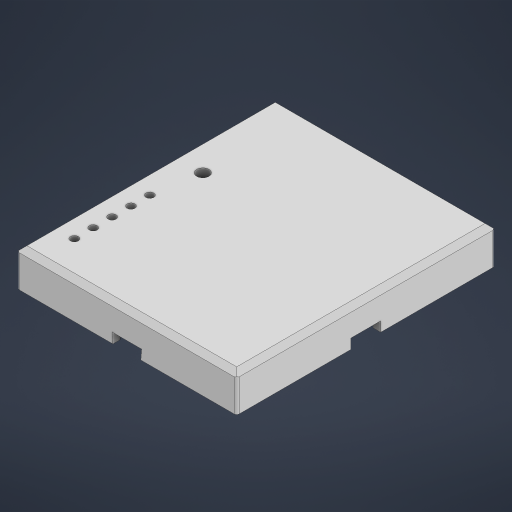
# Autodesk Inventor part: enclosure3_top
Saved by Autodesk Inventor 2023 (Build 270158000, 158)
## iProperties
Created: 2022-05-05
Part Number: enclosure3_top
Material: Generic
Document SubType Name: Modeling
Designer: Haroon Nawaz
Density: 1 g/cm^3
Appearance: Default
Author: Haroon Nawaz
Autodesk Inventor part; units mm, degrees
note: some values were not read from the file. Chosen so that the rebuilt part matches the saved one: direction of "Emboss2".
ref_plane "YZ Plane" through (0, 0, 0) normal (1, 0, 0) x (0, 1, 0)
ref_plane "XZ Plane" through (0, 0, 0) normal (0, 1, 0) x (-1, 0, 0)
ref_plane "XY Plane" through (0, 0, 0) normal (0, 0, 1) x (1, 0, 0)
sketch "Sketch1" plane through (0, 0, 0) normal (0, 1, 0) x (-1, 0, 0)
  line L0 (0, 0) -> (44.4, 0)
  line L1 (44.4, 0) -> (44.4, -52.2)
  line L2 (44.4, -52.2) -> (0, -52.2)
  line L3 (0, -52.2) -> (0, 0)
  dimension "d2" = 44.4
  dimension "d3" = 52.2
  constraints: 8 end point, 2 parallel, 1 horizontal, 1 perpendicular
  measures "d2" distance of L1.end L2.end
  measures "d3" distance of L0.end L1.end
extrude "Extrusion1" add sketch "Sketch1" along normal blind 7.5
shell "Shell1" thickness 1.5 removed faces 1 at (-14.8, 0, -17.4)
chamfer "Chamfer1" distance 1 angle 45 5 edges at (0, 7.5, -26.1) (-22.2, 7.5, 0) (-22.2, 7.5, -52.2) (-44.4, 7.5, -26.1) (-42.9, 3, -50.7)
sketch "Sketch3" plane through (0, 7.5, 0) normal (0, 1, 0) x (1, 0, 0)
  line L0 (-44.4, 52.2) -> (-44.4, 31.531)
  line L1 (-44.4, 52.2) -> (-44.4, 0) projected
  line L2 (-44.4, 31.531) -> (-38.38, 31.531)
  point P0 (0, 0)
  point P1 (-44.4, 51.45)
  point P2 (-44.4, 0.75)
  dimension "d26" = 20.669
  dimension "d27" = 6.02
  constraints: 4 end point, 1 coincident, 1 horizontal, 1 point on line
  measures "d26" distance of L0.start L0.end
  measures "d27" distance of L0.end L2.end
hole "Hole1" at (-38.38, 7.5, -31.531) direction (0, -1, 0) diameter 2.5 depth 3 tip angle 118
fillet "Fillet1" radius 0.5 4 edges at (0, 3.25, -52.2) (0, 3.25, 0) (-44.4, 3.25, -52.2) (-44.4, 3.25, 0)
sketch "Sketch4" plane through (-1.5, 6, -50.7) normal (0, -1, 0) x (1, 0, 0)
  circle A0 centre (-36.88, 19.169) radius 1.25 projected
  circle A1 centre (-36.88, 19.169) radius 1.5
  circle A2 centre (-36.88, 19.169) radius 1.125
  point P0 (1.5, 50.7)
  dimension "d36" = 3
  dimension "d40" = 2.25
  constraints: 2 centre point, 2 coincident
  measures "d36" diameter of A1
  measures "d40" diameter of A2
extrude "Extrusion3" add sketch "Sketch4" along normal blind 2.4 contours A1
fillet "Fillet2" radius 0.5 1 edges at (-39.88, 6, -31.531)
sketch "Sketch5" plane through (0, 7.5, 0) normal (0, 1, 0) x (1, 0, 0)
  line L0 (-44.3114, 52.075) -> (-44.3114, 22.635)
  line L1 (-44.4, 51.7) -> (-44.4, 0.5) projected
  line L2 (-44.3114, 52.075) -> (-14.8714, 52.075) construction
  line L3 (0, 0.5) -> (0, 51.7) projected
  point P0 (0, 0)
  point P1 (-44.4, 0)
  point P2 (-39.8266, 22.26)
  point P3 (-39.8266, 18.45)
  point P4 (-39.8266, 14.64)
  point P5 (-39.8266, 10.83)
  point P6 (-39.8266, 7.02)
  dimension "d41" = 29.44
  dimension "d42" = 90
  dimension "d46" = 3.81
  dimension "d58" = 4.5734
  dimension "d81" = 39.8266
  constraints: 4 end point, 1 horizontal, 1 parallel, 1 perpendicular, 1 vertical, 4 other
  measures "d41" distance of L0.start L0.end
  measures "d42" angle of L0 L2
  measures "d46" distance of point (-39.827, 22.26) point (-39.827, 18.45)
  measures "d58" distance from line of L1 point (-39.827, 22.26)
  measures "d81" distance from line of point (-39.827, 22.26) L3
hole "Hole2" at (-39.8266, 7.5, -22.26) at (-39.8266, 7.5, -18.45) at (-39.8266, 7.5, -14.64) at (-39.8266, 7.5, -10.83) at (-39.8266, 7.5, -7.02) direction (0, -1, 0) diameter 1.6 depth 3 tip angle 118
sketch "Sketch6" plane through (-0.5, 0, -52.2) normal (0, 0, -1) x (-1, 0, 0)
  line L0 (-0.5, 0) -> (1.82, 0)
  line L1 (-0.5, 0) -> (33.3, 0)
  line L2 (42.4, 0) -> (1, 0) projected
  line L3 (1.82, 0) -> (33.3, 0)
  line L4 (33.3, 0) -> (33.3, 3.175)
  line L5 (33.3, 3.175) -> (1.82, 3.175)
  line L6 (1.82, 3.175) -> (1.82, 0)
  point P0 (41.9, 0)
  dimension "d59" = 2.32
  dimension "d60" = 33.8
  dimension "d61" = 3.175
  constraints: 12 end point, 2 horizontal, 2 parallel, 1 perpendicular, 1 point on line
  measures "d59" distance of L0.start L0.end
  measures "d60" distance of L0.start L1.end
  measures "d61" distance of L3.end L4.end
extrude "Extrusion4" cut sketch "Sketch6" against normal blind 1.5
sketch "Sketch8" plane through (-1.5, 6, -50.7) normal (0, -1, 0) x (1, 0, 0)
  line L0 (-18.1366, 47.9399) -> (24.8957, 47.9399) construction
  line L1 (24.8957, 47.9399) -> (24.8957, 43.6819) construction
  line L2 (24.8957, 43.6819) -> (-18.1366, 43.6819) construction
  line L3 (-18.1366, 43.6819) -> (-18.1366, 47.9399) construction
  line L4 (-16.6442, 44.4831) -> (-18.0503, 44.4831)
  line L5 (-18.0503, 44.4831) -> (-18.0503, 44.6455)
  spline S0 degree 2 poles (-18.0503, 44.6455) (-17.9919, 44.6506) (-17.8828, 44.6633) (-17.8396, 44.6785) knots 0 0 0 1 2 2 2
  spline S1 degree 2 poles (-17.8396, 44.6785) (-17.766, 44.7064) (-17.7152, 44.8054) (-17.7152, 44.8891) knots 0 0 0 1 2 2 2
  line L6 (-17.7152, 44.8891) -> (-17.7152, 47.3637)
  spline S2 degree 2 poles (-17.7152, 47.3637) (-17.7152, 47.45) (-17.7838, 47.5947) (-17.8421, 47.6328) knots 0 0 0 1 2 2 2
  spline S3 degree 2 poles (-17.8421, 47.6328) (-17.8878, 47.6607) (-18.068, 47.714) (-18.1366, 47.7191) knots 0 0 0 1 2 2 2
  line L7 (-18.1366, 47.7191) -> (-18.1366, 47.8815)
  line L8 (-18.1366, 47.8815) -> (-17.0122, 47.9399)
  line L9 (-17.0122, 47.9399) -> (-16.9792, 47.9043)
  line L10 (-16.9792, 47.9043) -> (-16.9792, 44.9171)
  spline S4 degree 2 poles (-16.9792, 44.9171) (-16.9792, 44.8358) (-16.9208, 44.7318) (-16.8549, 44.7039) knots 0 0 0 1 2 2 2
  spline S5 degree 2 poles (-16.8549, 44.7039) (-16.8117, 44.6836) (-16.7127, 44.6531) (-16.6442, 44.6455) knots 0 0 0 1 2 2 2
  line L11 (-16.6442, 44.6455) -> (-16.6442, 44.4831)
  spline S6 degree 2 poles (-14.0326, 45.0186) (-14.1112, 44.8891) (-14.332, 44.6633) (-14.4716, 44.5846) knots 0 0 0 1 2 2 2
  spline S7 degree 2 poles (-14.4716, 44.5846) (-14.6214, 44.4983) (-14.9285, 44.412) (-15.1265, 44.412) knots 0 0 0 1 2 2 2
  spline S8 degree 2 poles (-15.1265, 44.412) (-15.4589, 44.412) (-15.9386, 44.5998) (-16.096, 44.7572) knots 0 0 0 1 2 2 2
  spline S9 degree 2 poles (-16.096, 44.7572) (-16.2508, 44.9171) (-16.4056, 45.3485) (-16.4056, 45.5998) knots 0 0 0 1 2 2 2
  spline S10 degree 2 poles (-16.4056, 45.5998) (-16.4056, 45.8282) (-16.2381, 46.247) (-16.0833, 46.4094) knots 0 0 0 1 2 2 2
  spline S11 degree 2 poles (-16.0833, 46.4094) (-15.931, 46.5693) (-15.4691, 46.7648) (-15.1848, 46.7648) knots 0 0 0 1 2 2 2
  spline S12 degree 2 poles (-15.1848, 46.7648) (-14.8701, 46.7648) (-14.4691, 46.6125) (-14.3371, 46.478) knots 0 0 0 1 2 2 2
  spline S13 degree 2 poles (-14.3371, 46.478) (-14.2102, 46.3511) (-14.0935, 46.0059) (-14.0935, 45.8155) knots 0 0 0 1 2 2 2
  line L12 (-14.0935, 45.8155) -> (-14.0935, 45.6709)
  line L13 (-14.0935, 45.6709) -> (-15.6036, 45.6709)
  spline S14 degree 2 poles (-15.6036, 45.6709) (-15.6036, 45.2115) (-15.2508, 44.7343) (-14.865, 44.7343) knots 0 0 0 1 2 2 2
  spline S15 degree 2 poles (-14.865, 44.7343) (-14.6569, 44.7343) (-14.3219, 44.9653) (-14.2026, 45.1404) knots 0 0 0 1 2 2 2
  line L14 (-14.2026, 45.1404) -> (-14.0326, 45.0186)
  spline S16 degree 2 poles (-14.8853, 45.8688) (-14.8853, 46.0008) (-14.9133, 46.2825) (-14.9463, 46.3714) knots 0 0 0 1 2 2 2
  spline S17 degree 2 poles (-14.9463, 46.3714) (-14.9843, 46.478) (-15.1163, 46.5846) (-15.2153, 46.5846) knots 0 0 0 1 2 2 2
  spline S18 degree 2 poles (-15.2153, 46.5846) (-15.3879, 46.5846) (-15.5934, 46.2368) (-15.6036, 45.8587) knots 0 0 0 1 2 2 2
  line L15 (-15.6036, 45.8587) -> (-14.8853, 45.8688)
  line L16 (-10.157, 46.445) -> (-10.6494, 46.445)
  spline S19 degree 2 poles (-10.6494, 46.445) (-10.5605, 46.3485) (-10.4742, 46.1302) (-10.4742, 46.011) knots 0 0 0 1 2 2 2
  spline S20 degree 2 poles (-10.4742, 46.011) (-10.4742, 45.8587) (-10.6392, 45.5871) (-10.7737, 45.5033) knots 0 0 0 1 2 2 2
  spline S21 degree 2 poles (-10.7737, 45.5033) (-10.9082, 45.4171) (-11.2763, 45.3181) (-11.4895, 45.3181) knots 0 0 0 1 2 2 2
  line L17 (-11.4895, 45.3181) -> (-11.8549, 45.3181)
  spline S22 degree 2 poles (-11.8549, 45.3181) (-11.8803, 45.2978) (-11.9463, 45.2115) (-11.9463, 45.1709) knots 0 0 0 1 2 2 2
  spline S23 degree 2 poles (-11.9463, 45.1709) (-11.9463, 45.0719) (-11.7889, 44.9957) (-11.5834, 44.9907) knots 0 0 0 1 2 2 2
  spline S24 degree 2 poles (-11.5834, 44.9907) (-11.3803, 44.9856) (-10.9666, 44.9627) (-10.8778, 44.9602) knots 0 0 0 1 2 2 2
  spline S25 degree 2 poles (-10.8778, 44.9602) (-10.7483, 44.9526) (-10.492, 44.8612) (-10.3981, 44.7876) knots 0 0 0 1 2 2 2
  spline S26 degree 2 poles (-10.3981, 44.7876) (-10.2966, 44.7089) (-10.1621, 44.4653) (-10.1621, 44.3079) knots 0 0 0 1 2 2 2
  spline S27 degree 2 poles (-10.1621, 44.3079) (-10.1621, 44.1379) (-10.3245, 43.8384) (-10.492, 43.7293) knots 0 0 0 1 2 2 2
  spline S28 degree 2 poles (-10.492, 43.7293) (-10.6697, 43.6151) (-11.162, 43.4907) (-11.525, 43.4907) knots 0 0 0 1 2 2 2
  spline S29 degree 2 poles (-11.525, 43.4907) (-12.1113, 43.4907) (-12.7229, 43.7775) (-12.7229, 44.0617) knots 0 0 0 1 2 2 2
  spline S30 degree 2 poles (-12.7229, 44.0617) (-12.7229, 44.2394) (-12.393, 44.4678) (-12.0478, 44.478) knots 0 0 0 1 2 2 2
  line L18 (-12.0478, 44.478) -> (-12.0478, 44.5059)
  spline S31 degree 2 poles (-12.0478, 44.5059) (-12.2534, 44.5744) (-12.4818, 44.8029) (-12.4818, 44.9551) knots 0 0 0 1 2 2 2
  spline S32 degree 2 poles (-12.4818, 44.9551) (-12.4818, 45.049) (-12.3905, 45.1785) (-12.3194, 45.2292) knots 0 0 0 1 2 2 2
  spline S33 degree 2 poles (-12.3194, 45.2292) (-12.2559, 45.2699) (-12.0757, 45.3308) (-12.0174, 45.3485) knots 0 0 0 1 2 2 2
  line L19 (-12.0174, 45.3485) -> (-12.0174, 45.3739)
  spline S34 degree 2 poles (-12.0174, 45.3739) (-12.3169, 45.4856) (-12.6011, 45.8079) (-12.6011, 46.0389) knots 0 0 0 1 2 2 2
  spline S35 degree 2 poles (-12.6011, 46.0389) (-12.6011, 46.3663) (-11.9971, 46.7597) (-11.5326, 46.7597) knots 0 0 0 1 2 2 2
  spline S36 degree 2 poles (-11.5326, 46.7597) (-11.3803, 46.7597) (-11.0961, 46.7089) (-11.0225, 46.6886) knots 0 0 0 1 2 2 2
  line L20 (-11.0225, 46.6886) -> (-10.157, 46.6886)
  line L21 (-10.157, 46.6886) -> (-10.157, 46.445)
  spline S37 degree 2 poles (-10.8321, 44.1455) (-10.8321, 44.2216) (-10.9159, 44.3714) (-11.0631, 44.4171) knots 0 0 0 1 2 2 2
  spline S38 degree 2 poles (-11.0631, 44.4171) (-11.1443, 44.4298) (-11.5098, 44.4399) (-11.8296, 44.4399) knots 0 0 0 1 2 2 2
  spline S39 degree 2 poles (-11.8296, 44.4399) (-11.9082, 44.3739) (-12.0123, 44.1886) (-12.0123, 44.0592) knots 0 0 0 1 2 2 2
  spline S40 degree 2 poles (-12.0123, 44.0592) (-12.0123, 44.0034) (-11.9488, 43.8689) (-11.8828, 43.813) knots 0 0 0 1 2 2 2
  spline S41 degree 2 poles (-11.8828, 43.813) (-11.8067, 43.747) (-11.6138, 43.6734) (-11.4209, 43.6734) knots 0 0 0 1 2 2 2
  spline S42 degree 2 poles (-11.4209, 43.6734) (-11.1341, 43.6734) (-10.8321, 43.8968) (-10.8321, 44.1455) knots 0 0 0 1 2 2 2
  spline S43 degree 2 poles (-11.2052, 46.0211) (-11.2052, 46.2825) (-11.3702, 46.5846) (-11.5428, 46.5846) knots 0 0 0 1 2 2 2
  spline S44 degree 2 poles (-11.5428, 46.5846) (-11.629, 46.5846) (-11.761, 46.5033) (-11.7991, 46.4247) knots 0 0 0 1 2 2 2
  spline S45 degree 2 poles (-11.7991, 46.4247) (-11.8372, 46.3485) (-11.8651, 46.1455) (-11.8651, 46.0389) knots 0 0 0 1 2 2 2
  spline S46 degree 2 poles (-11.8651, 46.0389) (-11.8651, 45.7952) (-11.695, 45.483) (-11.5377, 45.483) knots 0 0 0 1 2 2 2
  spline S47 degree 2 poles (-11.5377, 45.483) (-11.3778, 45.483) (-11.2052, 45.7648) (-11.2052, 46.0211) knots 0 0 0 1 2 2 2
  spline S48 degree 2 poles (-7.619, 45.0186) (-7.6976, 44.8891) (-7.9184, 44.6633) (-8.058, 44.5846) knots 0 0 0 1 2 2 2
  spline S49 degree 2 poles (-8.058, 44.5846) (-8.2078, 44.4983) (-8.5149, 44.412) (-8.7128, 44.412) knots 0 0 0 1 2 2 2
  spline S50 degree 2 poles (-8.7128, 44.412) (-9.0453, 44.412) (-9.525, 44.5998) (-9.6824, 44.7572) knots 0 0 0 1 2 2 2
  spline S51 degree 2 poles (-9.6824, 44.7572) (-9.8372, 44.9171) (-9.992, 45.3485) (-9.992, 45.5998) knots 0 0 0 1 2 2 2
  spline S52 degree 2 poles (-9.992, 45.5998) (-9.992, 45.8282) (-9.8245, 46.247) (-9.6697, 46.4094) knots 0 0 0 1 2 2 2
  spline S53 degree 2 poles (-9.6697, 46.4094) (-9.5174, 46.5693) (-9.0555, 46.7648) (-8.7712, 46.7648) knots 0 0 0 1 2 2 2
  spline S54 degree 2 poles (-8.7712, 46.7648) (-8.4565, 46.7648) (-8.0555, 46.6125) (-7.9235, 46.478) knots 0 0 0 1 2 2 2
  spline S55 degree 2 poles (-7.9235, 46.478) (-7.7966, 46.3511) (-7.6799, 46.0059) (-7.6799, 45.8155) knots 0 0 0 1 2 2 2
  line L22 (-7.6799, 45.8155) -> (-7.6799, 45.6709)
  line L23 (-7.6799, 45.6709) -> (-9.19, 45.6709)
  spline S56 degree 2 poles (-9.19, 45.6709) (-9.19, 45.2115) (-8.8372, 44.7343) (-8.4514, 44.7343) knots 0 0 0 1 2 2 2
  spline S57 degree 2 poles (-8.4514, 44.7343) (-8.2433, 44.7343) (-7.9083, 44.9653) (-7.789, 45.1404) knots 0 0 0 1 2 2 2
  line L24 (-7.789, 45.1404) -> (-7.619, 45.0186)
  spline S58 degree 2 poles (-8.4717, 45.8688) (-8.4717, 46.0008) (-8.4997, 46.2825) (-8.5326, 46.3714) knots 0 0 0 1 2 2 2
  spline S59 degree 2 poles (-8.5326, 46.3714) (-8.5707, 46.478) (-8.7027, 46.5846) (-8.8017, 46.5846) knots 0 0 0 1 2 2 2
  spline S60 degree 2 poles (-8.8017, 46.5846) (-8.9743, 46.5846) (-9.1798, 46.2368) (-9.19, 45.8587) knots 0 0 0 1 2 2 2
  line L25 (-9.19, 45.8587) -> (-8.4717, 45.8688)
  spline S61 degree 2 poles (-6.3702, 44.4069) (-6.5885, 44.4069) (-7.0022, 44.5364) (-7.1164, 44.6074) knots 0 0 0 1 2 2 2
  line L26 (-7.1164, 44.6074) -> (-7.1824, 44.4551)
  line L27 (-7.1824, 44.4551) -> (-7.3575, 44.4551)
  line L28 (-7.3575, 44.4551) -> (-7.3855, 45.2876)
  line L29 (-7.3855, 45.2876) -> (-7.223, 45.2876)
  spline S62 degree 2 poles (-7.223, 45.2876) (-7.19, 45.1861) (-7.0327, 44.9348) (-6.9312, 44.8333) knots 0 0 0 1 2 2 2
  spline S63 degree 2 poles (-6.9312, 44.8333) (-6.8271, 44.7343) (-6.5555, 44.5947) (-6.4032, 44.5947) knots 0 0 0 1 2 2 2
  spline S64 degree 2 poles (-6.4032, 44.5947) (-6.1977, 44.5947) (-5.9997, 44.7521) (-5.9997, 44.9196) knots 0 0 0 1 2 2 2
  spline S65 degree 2 poles (-5.9997, 44.9196) (-5.9997, 45.0084) (-6.0885, 45.1252) (-6.1672, 45.1658) knots 0 0 0 1 2 2 2
  spline S66 degree 2 poles (-6.1672, 45.1658) (-6.2535, 45.2115) (-6.4616, 45.2749) (-6.6139, 45.3181) knots 0 0 0 1 2 2 2
  spline S67 degree 2 poles (-6.6139, 45.3181) (-6.7662, 45.3638) (-6.9819, 45.4551) (-7.0987, 45.5541) knots 0 0 0 1 2 2 2
  spline S68 degree 2 poles (-7.0987, 45.5541) (-7.1976, 45.6404) (-7.3195, 45.8866) (-7.3195, 46.0566) knots 0 0 0 1 2 2 2
  spline S69 degree 2 poles (-7.3195, 46.0566) (-7.3195, 46.3714) (-6.7916, 46.7597) (-6.3626, 46.7597) knots 0 0 0 1 2 2 2
  spline S70 degree 2 poles (-6.3626, 46.7597) (-6.1596, 46.7597) (-5.817, 46.6759) (-5.7002, 46.6277) knots 0 0 0 1 2 2 2
  line L30 (-5.7002, 46.6277) -> (-5.6545, 46.7597)
  line L31 (-5.6545, 46.7597) -> (-5.4845, 46.7597)
  line L32 (-5.4845, 46.7597) -> (-5.4489, 45.9983)
  line L33 (-5.4489, 45.9983) -> (-5.6063, 45.9983)
  spline S71 degree 2 poles (-5.6063, 45.9983) (-5.685, 46.2292) (-6.0631, 46.5668) (-6.2814, 46.5668) knots 0 0 0 1 2 2 2
  spline S72 degree 2 poles (-6.2814, 46.5668) (-6.454, 46.5668) (-6.6494, 46.4247) (-6.6494, 46.2978) knots 0 0 0 1 2 2 2
  spline S73 degree 2 poles (-6.6494, 46.2978) (-6.6494, 46.1277) (-6.3626, 45.9754) (-6.1038, 45.9094) knots 0 0 0 1 2 2 2
  spline S74 degree 2 poles (-6.1038, 45.9094) (-5.7053, 45.8054) (-5.3347, 45.4501) (-5.3347, 45.1759) knots 0 0 0 1 2 2 2
  spline S75 degree 2 poles (-5.3347, 45.1759) (-5.3347, 44.8079) (-5.9083, 44.4069) (-6.3702, 44.4069) knots 0 0 0 1 2 2 2
  spline S76 degree 2 poles (-3.4008, 44.5846) (-3.5429, 44.5237) (-3.8703, 44.4221) (-4.1038, 44.4221) knots 0 0 0 1 2 2 2
  spline S77 degree 2 poles (-4.1038, 44.4221) (-4.4515, 44.4221) (-4.7891, 44.7622) (-4.7891, 45.0744) knots 0 0 0 1 2 2 2
  line L34 (-4.7891, 45.0744) -> (-4.7891, 46.445)
  line L35 (-4.7891, 46.445) -> (-5.1901, 46.445)
  line L36 (-5.1901, 46.445) -> (-5.1901, 46.6886)
  line L37 (-5.1901, 46.6886) -> (-4.7789, 46.6886)
  line L38 (-4.7789, 46.6886) -> (-4.7789, 47.3663)
  line L39 (-4.7789, 47.3663) -> (-4.0581, 47.3663)
  line L40 (-4.0581, 47.3663) -> (-4.0581, 46.6886)
  line L41 (-4.0581, 46.6886) -> (-3.4287, 46.6886)
  line L42 (-3.4287, 46.6886) -> (-3.4287, 46.445)
  line L43 (-3.4287, 46.445) -> (-4.053, 46.445)
  line L44 (-4.053, 46.445) -> (-4.053, 45.2242)
  spline S78 degree 2 poles (-4.053, 45.2242) (-4.053, 44.9627) (-3.9084, 44.7445) (-3.718, 44.7445) knots 0 0 0 1 2 2 2
  spline S79 degree 2 poles (-3.718, 44.7445) (-3.6596, 44.7445) (-3.4439, 44.7622) (-3.4008, 44.7724) knots 0 0 0 1 2 2 2
  line L45 (-3.4008, 44.7724) -> (-3.4008, 44.5846)
  spline S80 degree 2 poles (-0.8424, 45.0186) (-0.9211, 44.8891) (-1.1419, 44.6633) (-1.2815, 44.5846) knots 0 0 0 1 2 2 2
  spline S81 degree 2 poles (-1.2815, 44.5846) (-1.4312, 44.4983) (-1.7383, 44.412) (-1.9363, 44.412) knots 0 0 0 1 2 2 2
  spline S82 degree 2 poles (-1.9363, 44.412) (-2.2688, 44.412) (-2.7485, 44.5998) (-2.9058, 44.7572) knots 0 0 0 1 2 2 2
  spline S83 degree 2 poles (-2.9058, 44.7572) (-3.0607, 44.9171) (-3.2155, 45.3485) (-3.2155, 45.5998) knots 0 0 0 1 2 2 2
  spline S84 degree 2 poles (-3.2155, 45.5998) (-3.2155, 45.8282) (-3.048, 46.247) (-2.8931, 46.4094) knots 0 0 0 1 2 2 2
  spline S85 degree 2 poles (-2.8931, 46.4094) (-2.7409, 46.5693) (-2.2789, 46.7648) (-1.9947, 46.7648) knots 0 0 0 1 2 2 2
  spline S86 degree 2 poles (-1.9947, 46.7648) (-1.68, 46.7648) (-1.279, 46.6125) (-1.147, 46.478) knots 0 0 0 1 2 2 2
  spline S87 degree 2 poles (-1.147, 46.478) (-1.0201, 46.3511) (-0.9033, 46.0059) (-0.9033, 45.8155) knots 0 0 0 1 2 2 2
  line L46 (-0.9033, 45.8155) -> (-0.9033, 45.6709)
  line L47 (-0.9033, 45.6709) -> (-2.4135, 45.6709)
  spline S88 degree 2 poles (-2.4135, 45.6709) (-2.4135, 45.2115) (-2.0607, 44.7343) (-1.6749, 44.7343) knots 0 0 0 1 2 2 2
  spline S89 degree 2 poles (-1.6749, 44.7343) (-1.4668, 44.7343) (-1.1318, 44.9653) (-1.0125, 45.1404) knots 0 0 0 1 2 2 2
  line L48 (-1.0125, 45.1404) -> (-0.8424, 45.0186)
  spline S90 degree 2 poles (-1.6952, 45.8688) (-1.6952, 46.0008) (-1.7231, 46.2825) (-1.7561, 46.3714) knots 0 0 0 1 2 2 2
  spline S91 degree 2 poles (-1.7561, 46.3714) (-1.7942, 46.478) (-1.9262, 46.5846) (-2.0251, 46.5846) knots 0 0 0 1 2 2 2
  spline S92 degree 2 poles (-2.0251, 46.5846) (-2.1977, 46.5846) (-2.4033, 46.2368) (-2.4135, 45.8587) knots 0 0 0 1 2 2 2
  line L49 (-2.4135, 45.8587) -> (-1.6952, 45.8688)
  point P0 (1.5, 50.7)
  dimension "d2" = 44.4
  dimension "d3" = 52.2
  constraints: 2 other
emboss "Emboss2" sketch "Sketch8" operation cut depth 0.7 direction (0, 1, 0)
sketch "Sketch9" plane through (0, 0, -0.5) normal (1, 0, 0) x (0, 0, -1)
  line L0 (-0.5, 6.5) -> (-0.5, 0) projected
  line L1 (-0.5, 0) -> (25.6, 0)
  line L2 (51.7, 3.175) -> (51.7, 0) projected
  line L3 (22.6, -2) -> (28.6, -2)
  line L4 (28.6, -2) -> (28.6, 2)
  line L5 (28.6, 2) -> (22.6, 2)
  line L6 (22.6, 2) -> (22.6, -2)
  line L7 (22.6, -2) -> (28.6, 2) construction
  line L8 (28.6, -2) -> (22.6, 2) construction
  dimension "d71" = 26.1
  dimension "d72" = 6
  dimension "d73" = 4
  constraints: 14 end point, 2 midpoint, 2 parallel, 2 perpendicular, 1 horizontal
  measures "d71" distance of L0.end L1.end
  measures "d72" distance of L5.end L4.end
  measures "d73" distance of L4.end L3.end
extrude "Extrusion5" cut sketch "Sketch9" against normal through all
sketch "Sketch10" plane through (-43.9, 0, 0) normal (0, 0, 1) x (1, 0, 0)
  line L0 (-0.5, 6.5) -> (-0.5, 0) projected
  line L1 (-0.5, 0) -> (21.7, 0)
  line L2 (18.7, -2) -> (24.7, -2)
  line L3 (24.7, -2) -> (24.7, 2)
  line L4 (24.7, 2) -> (18.7, 2)
  line L5 (18.7, 2) -> (18.7, -2)
  line L6 (18.7, -2) -> (24.7, 2) construction
  line L7 (24.7, -2) -> (18.7, 2) construction
  line L8 (1, 0) -> (42.4, 0) projected
  line L9 (18.7, 0) -> (18.875, 0)
  line L10 (18.875, 0) -> (18.7, 2)
  line L11 (24.7, 0) -> (24.525, 0)
  line L12 (24.525, 0) -> (24.7, 2)
  point P0 (43.9, 0)
  dimension "d76" = 22.2
  dimension "d77" = 6
  dimension "d78" = 4
  dimension "d82" = 0.175
  dimension "d83" = 0.175
  constraints: 22 end point, 4 midpoint, 4 point on line, 2 horizontal, 2 parallel, 1 perpendicular
  measures "d76" distance of L0.end L1.end
  measures "d77" distance of L4.end L3.end
  measures "d78" distance of L3.end L2.end
  measures "d82" distance of L9.start L9.end
  measures "d83" distance of L11.start L11.end
extrude "Extrusion6" cut sketch "Sketch10" against normal blind 10 contours L1 L8 L3 L2 L5 | L10 L4 L12 L8 L1
equation "\"d2\" = d0"
equation "\"d3\" = d1"
equation "\"d35\" = outside_fillet"
equation "\"d0\" = 44.4"
equation "\"d1\" = 52.2"
equation "\"outside_fillet\" = 0.5"
body "Solid1"
